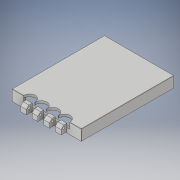
# Autodesk Inventor part: Hand Base Summ
Saved by Autodesk Inventor 2017 (Build 210142000, 142)
## iProperties
Created: 2018-11-20
Part Number: Hand Base Summ
Material: Generic
Document SubType Name: Modeling
Designer: S346795925
Density: 1 g/cm^3
Appearance: Default
Author: S346795925
Autodesk Inventor part; units mm, degrees
sketch "Sketch1" plane through (0, 0, 0) normal (0, 1, 0) x (-1, 0, 0)
  line L0 (0, 0) -> (-76.2, 0)
  line L1 (-76.2, 0) -> (-76.2, 101.6)
  line L2 (-76.2, 101.6) -> (0, 101.6)
  line L3 (0, 101.6) -> (0, 101.6)
  line L4 (0, 101.6) -> (0, 74.1605)
  line L5 (0, 74.1605) -> (0, 54.0859)
  line L6 (0, 54.0859) -> (0, 0)
  dimension "d0" = 76.2
  dimension "d1" = 101.6
  constraints: 14 end point, 2 parallel, 1 horizontal, 1 perpendicular, 1 vertical
  measures "d0" distance of L1.end L2.end
  measures "d1" distance of L0.end L1.end
extrude "Extrusion1" add sketch "Sketch1" along normal blind 25.4
shell "Shell1" thickness 2.54 removed faces 1 at (50.8, 0, 51.8953)
fillet "Fillet2" radius 0.3175 15 edges at (38.1, 25.4, 101.6) (76.2, 25.4, 50.8) (38.1, 25.4, 0) (0, 25.4, 50.8) (0, 12.7, 101.6) (76.2, 12.7, 101.6) (76.2, 12.7, 0) (0, 12.7, 0) (2.54, 22.86, 50.8) (2.54, 11.43, 99.06) (73.66, 11.43, 99.06) (73.66, 22.86, 50.8) (73.66, 11.43, 2.54) (38.1, 22.86, 2.54) (2.54, 11.43, 2.54)
sketch "Sketch3" plane through (0, 0, 0) normal (1, 0, 0) x (0, 1, 0)
  line L0 (12.065, 101.6) -> (18.415, 101.6) projected
  line L1 (25.0825, 101.6) -> (25.0825, 102.87)
  line L2 (0, 98.7425) -> (22.5425, 98.7425) projected
  line L3 (20.0025, 107.95) -> (8.5261, 107.95)
  line L4 (14.9225, 102.87) -> (14.9225, 101.6)
  line L5 (25.0825, 102.87) -> (20.0025, 107.95)
  circle A0 centre (20.0025, 104.902) radius 1.3208
  line L6 (25.0825, 101.6) -> (0, 101.6) projected
  line L7 (25.0825, 101.6) -> (14.9225, 101.6)
  line L8 (0, 101.6) -> (25.0825, 101.6) projected
  line L9 (14.9225, 102.87) -> (14.9225, 107.95)
  line L10 (8.5261, 107.95) -> (14.9225, 107.95)
  point P0 (0, 0)
  point P1 (25.0825, 107.95)
  dimension "d30" = 6.35
  dimension "d31" = 10.16
  dimension "d32" = 5.08
  dimension "d33" = 5.08
  dimension "d35" = 5.08
  dimension "d36" = 2.6416
  dimension "d37" = 3.302
  dimension "d46" = 5.08
  constraints: 14 end point, 4 perpendicular, 4 point on line, 1 centre point, 1 collinear, 1 vertical
  measures "d30" distance of L1.start point (25.082, 107.95)
  measures "d31" distance of point (25.082, 107.95) L9.end
  measures "d32" distance of L1.end point (25.082, 107.95)
  measures "d33" distance of L3.start point (25.082, 107.95)
  measures "d35" distance of L4.start L9.end
  measures "d36" diameter of A0
  measures "d37" distance from line of L6 A0.centre
  measures "d46" distance from line of L9 A0.centre
ref_plane "Work Plane1" through (15.875, 15.24, 101.6) normal (1, 0, 0) x (0, 1, 0)
ref_plane "Work Plane2" through (22.225, 15.24, 101.6) normal (1, 0, 0) x (0, 1, 0)
ref_plane "Work Plane3" through (28.575, 15.24, 101.6) normal (1, 0, 0) x (0, 1, 0)
ref_plane "Work Plane4" through (41.275, 15.24, 101.6) normal (1, 0, 0) x (0, 1, 0)
ref_plane "Work Plane5" through (53.975, 15.24, 101.6) normal (1, 0, 0) x (0, 1, 0)
ref_plane "Work Plane6" through (60.325, 15.24, 101.6) normal (1, 0, 0) x (0, 1, 0)
ref_plane "Work Plane7" through (47.625, 15.24, 101.6) normal (1, 0, 0) x (0, 1, 0)
ref_plane "Work Plane8" through (34.925, 15.24, 101.6) normal (1, 0, 0) x (0, 1, 0)
extrude "Extrusion3" add sketch "Sketch3" along normal up to surface (6.35 mm away) from surface at 15.875
extrude "Extrusion4" add sketch "Sketch3" along normal up to surface (6.35 mm away) from surface at 28.575
extrude "Extrusion5" add sketch "Sketch3" along normal up to surface (6.35 mm away) from surface at 41.275
extrude "Extrusion6" add sketch "Sketch3" along normal up to surface (6.35 mm away) from surface at 53.975
sketch "Sketch4" plane through (0, 25.4, 0) normal (0, 1, 0) x (1, 0, 0)
  line L0 (75.8825, -101.2825) -> (0.3175, -101.2825) projected
  circle A0 centre (19.05, -101.2825) radius 6.35
  line L1 (0.3175, -101.2825) -> (0.3175, -0.3175) projected
  line L2 (0, -101.2825) -> (0, -0.3175) projected
  line L3 (0, -0.3175) -> (0, -101.2825) projected
  circle A1 centre (31.75, -101.2825) radius 6.35
  circle A2 centre (44.45, -101.2825) radius 6.35
  circle A3 centre (57.15, -101.2825) radius 6.35
  point P0 (0, 0)
  dimension "d47" = 12.7
  dimension "d49" = 19.05
  dimension "d52" = 12.7
  constraints: 4 centre point, 1 horizontal, 1 point on line, 6 other
  measures "d47" diameter of A0
  measures "d49" distance from line of A0.centre L2
  measures "d52" distance of A0.centre A1.centre
extrude "Extrusion7" cut sketch "Sketch4" against normal blind 2.54
sketch "Sketch5" plane through (0.3175, 0, 101.6) normal (0, 0, 1) x (1, 0, 0)
  line L0 (73.025, 22.86) -> (2.54, 22.86) projected
  line L1 (12.3746, 22.86) -> (63.1746, 22.86)
  line L2 (63.1746, 22.86) -> (63.1746, 18.9945)
  line L3 (63.1746, 18.9945) -> (12.3746, 18.9945)
  line L4 (12.3746, 18.9945) -> (12.3746, 22.86)
  point P0 (-0.3175, 0)
  dimension "d59" = 50.8
  constraints: 8 end point, 2 parallel, 1 horizontal, 1 perpendicular, 1 point on line
  measures "d59" distance of L2.end L3.end
extrude "Extrusion8" cut sketch "Sketch5" against normal blind 3.81
sketch "Sketch6" plane through (0, 0, 0) normal (0, -1, 0) x (1, 0, 0)
  arc A0 (75.8825, 0) -> (76.2, 0.3175) centre (75.8825, 0.3175) ccw projected
  line L0 (76.2, 0.3175) -> (76.2, 101.2825) projected
  arc A1 (76.2, 101.2825) -> (75.8825, 101.6) centre (75.8825, 101.2825) ccw projected
  line L1 (75.8825, 101.6) -> (0.3175, 101.6) projected
  arc A2 (0.3175, 101.6) -> (0, 101.2825) centre (0.3175, 101.2825) ccw projected
  line L2 (0, 101.2825) -> (0, 0.3175) projected
  arc A3 (0, 0.3175) -> (0.3175, 0) centre (0.3175, 0.3175) ccw projected
  line L3 (0.3175, 0) -> (75.8825, 0) projected
  line L4 (73.66, 98.7425) -> (73.66, 2.8575) projected
  arc A4 (73.3425, 2.54) -> (73.66, 2.8575) centre (73.3425, 2.8575) ccw projected
  line L5 (73.3425, 2.54) -> (2.8575, 2.54) projected
  arc A5 (2.54, 2.8575) -> (2.8575, 2.54) centre (2.8575, 2.8575) ccw projected
  line L6 (2.54, 2.8575) -> (2.54, 98.7425) projected
  arc A6 (2.8575, 99.06) -> (2.54, 98.7425) centre (2.8575, 98.7425) ccw projected
  line L7 (2.8575, 99.06) -> (73.3425, 99.06) projected
  arc A7 (73.66, 98.7425) -> (73.3425, 99.06) centre (73.3425, 98.7425) ccw projected
  point P0 (0, 0)
extrude "Extrusion9" cut sketch "Sketch6" against normal blind 13.6525
equation "\"d33\" = d32"
equation "\"d35\" = d34"
equation "\"d34\" = d32"
body "Solid1"
